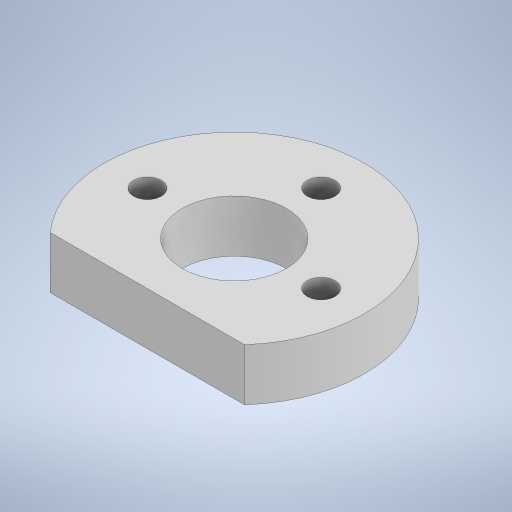
# Autodesk Inventor part: 射出_留め具3
Saved by Autodesk Inventor 2023 (Build 270158000, 158)
## iProperties
Created: 2022-05-03
Part Number: 射出_留め具3
Material: 一般
Document SubType Name: Modeling
Designer: yuta
Density: 1 g/cm^3
Appearance: 既定
Author: yuta
Autodesk Inventor part; units mm, degrees
ref_plane "YZ Plane" through (0, 0, 0) normal (1, 0, 0) x (0, 1, 0)
ref_plane "XZ Plane" through (0, 0, 0) normal (0, 1, 0) x (-1, 0, 0)
ref_plane "XY Plane" through (0, 0, 0) normal (0, 0, 1) x (1, 0, 0)
sketch "スケッチ1" plane through (0, 0, 0) normal (0, 1, 0) x (-1, 0, 0)
  circle A0 centre (0, 0) radius 15
  dimension "d0" = 30
  constraints: 1 centre point, 1 coincident
  measures "d0" diameter of A0
extrude "押し出し1" add sketch "スケッチ1" along normal blind 6
sketch "スケッチ2" plane through (0, 6, 0) normal (0, 1, 0) x (1, 0, 0)
  arc A0 (2.6833, -3.1) -> (-2.6833, -3.1) centre (0, 0) ccw
  line L0 (-2.6833, -3.1) -> (2.6833, -3.1)
  point P0 (0, -3.1)
  dimension "d3" = 8.2
  dimension "d4" = 3.1
  constraints: 2 end point, 2 point on circle, 1 centre point, 1 coincident, 1 horizontal
  measures "d3" diameter of A0
  measures "d4" distance of point (0, 0) point (0, -3.1)
extrude "押し出し2" cut sketch "スケッチ2" against normal blind 6
sketch "スケッチ3" plane through (0, 6, 0) normal (0, 1, 0) x (1, 0, 0)
  circle A0 centre (0, 0) radius 15 projected
  circle A1 centre (0, 0) radius 15 projected
  line L0 (-11.1803, -10) -> (11.1803, -10)
  arc A2 (-11.1803, -10) -> (11.1803, -10) centre (0, 0) ccw
  point P0 (0, -10)
  dimension "d7" = 10
  constraints: 4 point on circle, 2 end point, 1 centre point, 1 concentric, 1 horizontal
  measures "d7" distance of point (0, -10) A0.centre
extrude "押し出し3" cut sketch "スケッチ3" against normal blind 6 contours L0 A0 picked at (2.8264, -10.7912)
sketch "スケッチ4" plane through (0, 6, 0) normal (0, 1, 0) x (1, 0, 0)
  circle A0 centre (0, 0) radius 10 construction
  point P0 (-10, 0)
  point P1 (0, 10)
  point P2 (10, 0)
  dimension "d10" = 20
  constraints: 3 point on circle, 1 centre point, 1 coincident
  measures "d10" diameter of A0
hole "穴1" at (-10, 6, 0) at (0, 6, -10) at (10, 6, 0) direction (0, -1, 0) diameter 3.2 end through all
sketch "スケッチ5" plane through (0, 6, 0) normal (0, 1, 0) x (1, 0, 0)
  circle A0 centre (0, 0) radius 6
  dimension "d18" = 12
  constraints: 1 centre point, 1 coincident
  measures "d18" diameter of A0
extrude "押し出し4" cut sketch "スケッチ5" against normal blind 10
